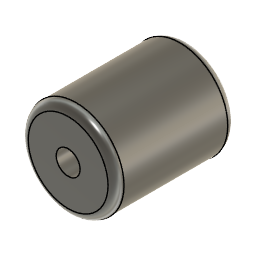
Roller (Autodesk Fusion 360 design; units mm, degrees)
part number: 2026-03-23-16-11-45-880
Autodesk Fusion 360 part; units mm, degrees
sketch "Sketch1" plane through (0, 0, 0) normal (0, 1, 0) x (1, 0, 0)
  circle A0 centre (0, 0) radius 15.24
  dimension "d1" = 30.48
  constraint coincident A0.centre origin
  measures "d1" diameter of A0
extrude "Extrude1" add sketch "Sketch1" along normal mid plane 38.1
fillet "Fillet1" radius 2.54 2 edges at (-14.2087, -19.05, -5.511) (-14.2087, 19.05, 5.511)
sketch "Sketch2" plane through (0, -19.05, 0) normal (0, -1, 0) x (1, 0, 0)
  circle A0 centre (0, 0) radius 12.7
  circle A1 centre (0, 0) radius 3.81
  dimension "d6" = 7.62
  constraint coincident A0.centre A1.centre
  measures "d6" diameter of A1
extrude "Extrude2" cut sketch "Sketch2" against normal through all contours A1
